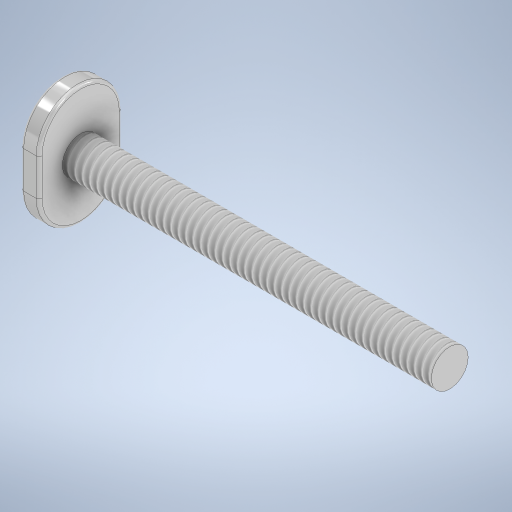
# Autodesk Inventor part: TeeBolt
Saved by Autodesk Inventor 2024 (Build 280153000, 153)
## iProperties
Created: 2023-06-18
Part Number: TeeBolt
Material: Generic
Document SubType Name: Modeling
Designer: 18179
Density: 1 g/cm^3
Appearance: Aluminum - Polished
Author: 18179
Autodesk Inventor part; units mm, degrees
ref_plane "YZ Plane" through (0, 0, 0) normal (1, 0, 0) x (0, 1, 0)
ref_plane "XZ Plane" through (0, 0, 0) normal (0, 1, 0) x (-1, 0, 0)
ref_plane "XY Plane" through (0, 0, 0) normal (0, 0, 1) x (1, 0, 0)
sketch "Sketch1" plane through (0, 0, 0) normal (1, 0, 0) x (0, 1, 0)
  line L0 (7.1501, 0) -> (13.4874, 0)
  line L1 (20.6375, -7.1501) -> (20.6375, -7.1501)
  line L2 (13.4874, -14.3002) -> (7.1501, -14.3002)
  line L3 (0, -7.1501) -> (0, -7.1501)
  arc A0 (20.6375, -7.1501) -> (13.4874, 0) centre (13.4874, -7.1501) ccw
  arc A1 (13.4874, -14.3002) -> (20.6375, -7.1501) centre (13.4874, -7.1501) ccw
  arc A2 (0, -7.1501) -> (7.1501, -14.3002) centre (7.1501, -7.1501) ccw
  arc A3 (7.1501, 0) -> (0, -7.1501) centre (7.1501, -7.1501) ccw
  point P0 (0, 0)
  point P1 (20.6375, -14.3002)
  point P2 (20.6375, 0)
  point P3 (0, -14.3002)
  dimension "d0" = 20.6375
  dimension "d1" = 14.3002
  dimension "d2" = 7.1501
  constraints: 8 end point, 8 point on circle, 8 point on line, 8 tangent, 4 centre point, 3 equal radius, 2 parallel, 1 horizontal, 1 perpendicular
  measures "d0" distance of point (20.637, -14.3) point (0, -14.3)
  measures "d1" distance of point (20.637, 0) point (20.637, -14.3)
  measures "d2" radius of A0
extrude "Extrusion1" add sketch "Sketch1" along normal blind 3.175
sketch "Sketch2" plane through (3.175, 0, 0) normal (1, 0, 0) x (0, 0, -1)
  line L0 (0, 13.4874) -> (0, 7.1501) projected
  line L1 (0, 10.3187) -> (14.3002, 10.3187)
  line L2 (14.3002, 7.1501) -> (14.3002, 13.4874) projected
  arc A0 (14.3002, 13.4874) -> (0, 13.4874) centre (7.1501, 13.4874) ccw projected
  arc A1 (0, 7.1501) -> (14.3002, 7.1501) centre (7.1501, 7.1501) ccw projected
  line L3 (7.1501, 13.4874) -> (7.1501, 7.1501)
  circle A2 centre (7.1501, 10.3187) radius 3.1686
  point P0 (0, 0)
  constraints: 4 end point, 3 midpoint, 1 vertical, 1 vertical alignment, 2 other
extrude "Extrusion2" add sketch "Sketch2" along normal blind 63.5 contours A2 L3 L1 | L1 L3 A2 | L3 A2 L1 | L1 A2 L3
thread "Thread1" size "1/4-20 UNC" class "2A" standard "ANSI Unified Screw Threads" full length
fillet "Fillet1" radius 0.508 8 edges at (3.175, 10.3187, 0) (3.175, 0, -7.1501) (3.175, 10.3187, -14.3002) (3.175, 20.6375, -7.1501) (0, 10.3187, 0) (0, 0, -7.1501) (0, 10.3187, -14.3002) (0, 20.6375, -7.1501)
body "Solid1"
